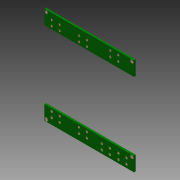
# Autodesk Inventor part: ui_pcb
Saved by Autodesk Inventor 2015 (Build 190159000, 159)
## iProperties
Created: 2014-10-14
Part Number: ui_pcb
Material: Generic
Document SubType Name: Modeling
Designer: Adam
Density: 1 g/cm^3
Appearance: Gold - Metal
Author: Adam
Autodesk Inventor part; units mm, degrees
ref_plane "YZ Plane" through (0, 0, 0) normal (1, 0, 0) x (0, 1, 0)
ref_plane "XZ Plane" through (0, 0, 0) normal (0, 1, 0) x (-1, 0, 0)
ref_plane "Work Plane1" through (0, 0, 0.25) normal (0, 0, 1) x (1, 0, 0)
sketch "Sketch1" plane through (0, 0, 0.25) normal (0, 0, 1) x (1, 0, 0)
  line L0 (4.3349, -0.3556) -> (4.6399, -0.3556) construction
  line L1 (4.6399, -0.3556) -> (4.6399, -1.0668) construction
  line L2 (4.6399, -1.0668) -> (4.3349, -1.0668) construction
  line L3 (4.3349, -1.0668) -> (4.3349, -0.3556) construction
  line L4 (-1.7314, -5.6515) -> (-2.0364, -5.6515) construction
  line L5 (-2.0364, -5.6515) -> (-2.0364, -4.9403) construction
  line L6 (-2.0364, -4.9403) -> (-1.7314, -4.9403) construction
  line L7 (-1.7314, -4.9403) -> (-1.7314, -5.6515) construction
  line L8 (-2.0364, -0.3556) -> (-1.7314, -0.3556) construction
  line L9 (-1.7314, -0.3556) -> (-1.7314, -1.0668) construction
  line L10 (-1.7314, -1.0668) -> (-2.0364, -1.0668) construction
  line L11 (-2.0364, -1.0668) -> (-2.0364, -0.3556) construction
  line L12 (4.3349, -4.9403) -> (4.6399, -4.9403) construction
  line L13 (4.6399, -4.9403) -> (4.6399, -5.6515) construction
  line L14 (4.6399, -5.6515) -> (4.3349, -5.6515) construction
  line L15 (4.3349, -5.6515) -> (4.3349, -4.9403) construction
  line L16 (27.1949, -0.3556) -> (27.4999, -0.3556) construction
  line L17 (27.4999, -0.3556) -> (27.4999, -1.0668) construction
  line L18 (27.4999, -1.0668) -> (27.1949, -1.0668) construction
  line L19 (27.1949, -1.0668) -> (27.1949, -0.3556) construction
  line L20 (21.1286, -5.6515) -> (20.8236, -5.6515) construction
  line L21 (20.8236, -5.6515) -> (20.8236, -4.9403) construction
  line L22 (20.8236, -4.9403) -> (21.1286, -4.9403) construction
  line L23 (21.1286, -4.9403) -> (21.1286, -5.6515) construction
  line L24 (20.8236, -0.3556) -> (21.1286, -0.3556) construction
  line L25 (21.1286, -0.3556) -> (21.1286, -1.0668) construction
  line L26 (21.1286, -1.0668) -> (20.8236, -1.0668) construction
  line L27 (20.8236, -1.0668) -> (20.8236, -0.3556) construction
  line L28 (27.1949, -4.9403) -> (27.4999, -4.9403) construction
  line L29 (27.4999, -4.9403) -> (27.4999, -5.6515) construction
  line L30 (27.4999, -5.6515) -> (27.1949, -5.6515) construction
  line L31 (27.1949, -5.6515) -> (27.1949, -4.9403) construction
  line L32 (46.3349, -2.665) -> (46.6399, -2.665) construction
  line L33 (46.6399, -2.665) -> (46.6399, -3.3762) construction
  line L34 (46.6399, -3.3762) -> (46.3349, -3.3762) construction
  line L35 (46.3349, -3.3762) -> (46.3349, -2.665) construction
  line L36 (40.2686, -7.9609) -> (39.9636, -7.9609) construction
  line L37 (39.9636, -7.9609) -> (39.9636, -7.2497) construction
  line L38 (39.9636, -7.2497) -> (40.2686, -7.2497) construction
  line L39 (40.2686, -7.2497) -> (40.2686, -7.9609) construction
  line L40 (39.9636, -2.665) -> (40.2686, -2.665) construction
  line L41 (40.2686, -2.665) -> (40.2686, -3.3762) construction
  line L42 (40.2686, -3.3762) -> (39.9636, -3.3762) construction
  line L43 (39.9636, -3.3762) -> (39.9636, -2.665) construction
  line L44 (46.3349, -7.2497) -> (46.6399, -7.2497) construction
  line L45 (46.6399, -7.2497) -> (46.6399, -7.9609) construction
  line L46 (46.6399, -7.9609) -> (46.3349, -7.9609) construction
  line L47 (46.3349, -7.9609) -> (46.3349, -7.2497) construction
  line L48 (60.3349, -2.665) -> (60.6399, -2.665) construction
  line L49 (60.6399, -2.665) -> (60.6399, -3.3762) construction
  line L50 (60.6399, -3.3762) -> (60.3349, -3.3762) construction
  line L51 (60.3349, -3.3762) -> (60.3349, -2.665) construction
  line L52 (54.2686, -7.9609) -> (53.9636, -7.9609) construction
  line L53 (53.9636, -7.9609) -> (53.9636, -7.2497) construction
  line L54 (53.9636, -7.2497) -> (54.2686, -7.2497) construction
  line L55 (54.2686, -7.2497) -> (54.2686, -7.9609) construction
  line L56 (53.9636, -2.665) -> (54.2686, -2.665) construction
  line L57 (54.2686, -2.665) -> (54.2686, -3.3762) construction
  line L58 (54.2686, -3.3762) -> (53.9636, -3.3762) construction
  line L59 (53.9636, -3.3762) -> (53.9636, -2.665) construction
  line L60 (60.3349, -7.2497) -> (60.6399, -7.2497) construction
  line L61 (60.6399, -7.2497) -> (60.6399, -7.9609) construction
  line L62 (60.6399, -7.9609) -> (60.3349, -7.9609) construction
  line L63 (60.3349, -7.9609) -> (60.3349, -7.2497) construction
  line L64 (4.3349, 66.082) -> (4.6399, 66.082) construction
  line L65 (4.6399, 66.082) -> (4.6399, 65.3708) construction
  line L66 (4.6399, 65.3708) -> (4.3349, 65.3708) construction
  line L67 (4.3349, 65.3708) -> (4.3349, 66.082) construction
  line L68 (-1.7314, 60.7861) -> (-2.0364, 60.7861) construction
  line L69 (-2.0364, 60.7861) -> (-2.0364, 61.4973) construction
  line L70 (-2.0364, 61.4973) -> (-1.7314, 61.4973) construction
  line L71 (-1.7314, 61.4973) -> (-1.7314, 60.7861) construction
  line L72 (-2.0364, 66.082) -> (-1.7314, 66.082) construction
  line L73 (-1.7314, 66.082) -> (-1.7314, 65.3708) construction
  line L74 (-1.7314, 65.3708) -> (-2.0364, 65.3708) construction
  line L75 (-2.0364, 65.3708) -> (-2.0364, 66.082) construction
  line L76 (4.3349, 61.4973) -> (4.6399, 61.4973) construction
  line L77 (4.6399, 61.4973) -> (4.6399, 60.7861) construction
  line L78 (4.6399, 60.7861) -> (4.3349, 60.7861) construction
  line L79 (4.3349, 60.7861) -> (4.3349, 61.4973) construction
  line L80 (27.1949, 66.082) -> (27.4999, 66.082) construction
  line L81 (27.4999, 66.082) -> (27.4999, 65.3708) construction
  line L82 (27.4999, 65.3708) -> (27.1949, 65.3708) construction
  line L83 (27.1949, 65.3708) -> (27.1949, 66.082) construction
  line L84 (21.1286, 60.7861) -> (20.8236, 60.7861) construction
  line L85 (20.8236, 60.7861) -> (20.8236, 61.4973) construction
  line L86 (20.8236, 61.4973) -> (21.1286, 61.4973) construction
  line L87 (21.1286, 61.4973) -> (21.1286, 60.7861) construction
  line L88 (20.8236, 66.082) -> (21.1286, 66.082) construction
  line L89 (21.1286, 66.082) -> (21.1286, 65.3708) construction
  line L90 (21.1286, 65.3708) -> (20.8236, 65.3708) construction
  line L91 (20.8236, 65.3708) -> (20.8236, 66.082) construction
  line L92 (27.1949, 61.4973) -> (27.4999, 61.4973) construction
  line L93 (27.4999, 61.4973) -> (27.4999, 60.7861) construction
  line L94 (27.4999, 60.7861) -> (27.1949, 60.7861) construction
  line L95 (27.1949, 60.7861) -> (27.1949, 61.4973) construction
  line L96 (47.2686, 63.0955) -> (46.9636, 63.0955) construction
  line L97 (46.9636, 63.0955) -> (46.9636, 63.8067) construction
  line L98 (46.9636, 63.8067) -> (47.2686, 63.8067) construction
  line L99 (47.2686, 63.8067) -> (47.2686, 63.0955) construction
  line L100 (53.3349, 68.3914) -> (53.6399, 68.3914) construction
  line L101 (53.6399, 68.3914) -> (53.6399, 67.6802) construction
  line L102 (53.6399, 67.6802) -> (53.3349, 67.6802) construction
  line L103 (53.3349, 67.6802) -> (53.3349, 68.3914) construction
  line L104 (53.6399, 63.0955) -> (53.3349, 63.0955) construction
  line L105 (53.3349, 63.0955) -> (53.3349, 63.8067) construction
  line L106 (53.3349, 63.8067) -> (53.6399, 63.8067) construction
  line L107 (53.6399, 63.8067) -> (53.6399, 63.0955) construction
  line L108 (47.2686, 67.6802) -> (46.9636, 67.6802) construction
  line L109 (46.9636, 67.6802) -> (46.9636, 68.3914) construction
  line L110 (46.9636, 68.3914) -> (47.2686, 68.3914) construction
  line L111 (47.2686, 68.3914) -> (47.2686, 67.6802) construction
  circle A0 centre (-2.0364, -5.2959) radius 0.5
  circle A1 centre (4.6399, -5.2959) radius 0.5
  circle A2 centre (4.6399, -0.7112) radius 0.5
  circle A3 centre (-2.0364, -0.7112) radius 0.5
  circle A4 centre (20.8236, -0.7112) radius 0.5
  circle A5 centre (20.8236, -5.2959) radius 0.5
  circle A6 centre (27.4999, -5.2959) radius 0.5
  circle A7 centre (27.4999, -0.7112) radius 0.5
  circle A8 centre (39.9636, -3.0206) radius 0.5
  circle A9 centre (39.9636, -7.6053) radius 0.5
  circle A10 centre (46.6399, -3.0206) radius 0.5
  circle A11 centre (46.6399, -7.6053) radius 0.5
  circle A12 centre (53.9636, -3.0206) radius 0.5
  circle A13 centre (53.9636, -7.6053) radius 0.5
  circle A14 centre (60.6399, -3.0206) radius 0.5
  circle A15 centre (60.6399, -7.6053) radius 0.5
  circle A16 centre (-2.0364, 65.7264) radius 0.5
  circle A17 centre (-2.0364, 61.1417) radius 0.5
  circle A18 centre (4.6399, 65.7264) radius 0.5
  circle A19 centre (4.6399, 61.1417) radius 0.5
  circle A20 centre (20.8236, 65.7264) radius 0.5
  circle A21 centre (20.8236, 61.1417) radius 0.5
  circle A22 centre (27.4999, 61.1417) radius 0.5
  circle A23 centre (27.4999, 65.7264) radius 0.5
  circle A24 centre (46.9636, 68.0358) radius 0.5
  circle A25 centre (46.9636, 63.4511) radius 0.5
  circle A26 centre (53.6399, 63.4511) radius 0.5
  circle A27 centre (53.6399, 68.0358) radius 0.5
  line L112 (66.7941, 1.6153) -> (-8.1906, 1.6153)
  line L113 (-8.1906, 1.6153) -> (-8.1906, -10.3847)
  line L114 (-8.1906, -10.3847) -> (66.7941, -10.3847)
  line L115 (66.7941, -10.3847) -> (66.7941, 1.6153)
  line L116 (-8.1906, 58.8153) -> (66.7941, 58.8153)
  line L117 (66.7941, 58.8153) -> (66.7941, 70.8153)
  line L118 (66.7941, 70.8153) -> (-8.1906, 70.8153)
  line L119 (-8.1906, 70.8153) -> (-8.1906, 58.8153)
  line L120 (33.3094, 57.8153) -> (-11.6662, 57.8153) construction
  line L121 (-11.6662, 2.6153) -> (63.2941, 2.6153) construction
  point P0 (0, 0)
  dimension "d1" = 1
  dimension "d4" = 12
  dimension "d5" = 12
  dimension "d10" = 1
  dimension "d11" = 1
  dimension "d12" = 74.9846
  dimension "d13" = 3.4756
  constraints: 240 end point, 58 horizontal, 56 vertical, 28 centre point, 28 midpoint, 27 equal radius, 4 parallel, 2 collinear, 2 perpendicular, 112 other
  measures "d1" diameter of A0
  measures "d4" distance between parallel lines of L112 L114
  measures "d5" distance between parallel lines of L116 L118
  measures "d10" distance between parallel lines of L120 L116
  measures "d11" distance between parallel lines of L121 L112
  measures "d12" distance of L117.end L118.end
  measures "d13" distance from line of L120.end L119
extrude "Extrusion1" add sketch "Sketch1" along normal blind 1.5
sketch "Sketch2" plane through (0, 0, 1.75) normal (0, 0, 1) x (1, 0, 0)
  circle A0 centre (-6.4906, -8.6847) radius 0.75 projected
  circle A1 centre (65.0941, -0.0847) radius 0.75 projected
  circle A2 centre (65.0941, 69.1153) radius 0.75 projected
  circle A3 centre (-6.4906, 69.1153) radius 0.75 projected
  point P0 (0, 0)
extrude "Extrusion2" cut sketch "Sketch2" against normal through all
sketch "Sketch3" plane through (0, 0, 1.75) normal (0, 0, 1) x (1, 0, 0)
  circle A0 centre (65.0941, 69.1153) radius 0.75 projected
  circle A1 centre (-6.4906, 69.1153) radius 0.75 projected
  circle A2 centre (53.6399, 68.0358) radius 0.5 projected
  circle A3 centre (53.6399, 63.4511) radius 0.5 projected
  circle A4 centre (46.9636, 63.4511) radius 0.5 projected
  circle A5 centre (46.9636, 68.0358) radius 0.5 projected
  circle A6 centre (27.4999, 65.7264) radius 0.5 projected
  circle A7 centre (27.4999, 61.1417) radius 0.5 projected
  circle A8 centre (20.8236, 61.1417) radius 0.5 projected
  circle A9 centre (20.8236, 65.7264) radius 0.5 projected
  circle A10 centre (4.6399, 61.1417) radius 0.5 projected
  circle A11 centre (4.6399, 65.7264) radius 0.5 projected
  circle A12 centre (-2.0364, 61.1417) radius 0.5 projected
  circle A13 centre (-2.0364, 65.7264) radius 0.5 projected
  line L0 (-8.1906, 58.8153) -> (66.7941, 58.8153) projected
  line L1 (66.7941, 58.8153) -> (66.7941, 70.8153) projected
  line L2 (66.7941, 70.8153) -> (-8.1906, 70.8153) projected
  line L3 (-8.1906, 70.8153) -> (-8.1906, 58.8153) projected
  circle A14 centre (-6.4906, -8.6847) radius 0.75 projected
  circle A15 centre (65.0941, -0.0847) radius 0.75 projected
  circle A16 centre (60.6399, -7.6053) radius 0.5 projected
  circle A17 centre (60.6399, -3.0206) radius 0.5 projected
  circle A18 centre (53.9636, -7.6053) radius 0.5 projected
  circle A19 centre (53.9636, -3.0206) radius 0.5 projected
  circle A20 centre (46.6399, -7.6053) radius 0.5 projected
  circle A21 centre (46.6399, -3.0206) radius 0.5 projected
  circle A22 centre (39.9636, -7.6053) radius 0.5 projected
  circle A23 centre (39.9636, -3.0206) radius 0.5 projected
  circle A24 centre (27.4999, -0.7112) radius 0.5 projected
  circle A25 centre (27.4999, -5.2959) radius 0.5 projected
  circle A26 centre (20.8236, -5.2959) radius 0.5 projected
  circle A27 centre (20.8236, -0.7112) radius 0.5 projected
  circle A28 centre (-2.0364, -0.7112) radius 0.5 projected
  circle A29 centre (4.6399, -0.7112) radius 0.5 projected
  circle A30 centre (4.6399, -5.2959) radius 0.5 projected
  circle A31 centre (-2.0364, -5.2959) radius 0.5 projected
  line L4 (66.7941, 1.6153) -> (-8.1906, 1.6153) projected
  line L5 (-8.1906, 1.6153) -> (-8.1906, -10.3847) projected
  line L6 (-8.1906, -10.3847) -> (66.7941, -10.3847) projected
  line L7 (66.7941, -10.3847) -> (66.7941, 1.6153) projected
  circle A32 centre (46.9636, 68.0358) radius 1
  circle A33 centre (46.9636, 63.4511) radius 1
  circle A34 centre (53.6399, 63.4511) radius 1
  circle A35 centre (53.6399, 68.0358) radius 1
  circle A36 centre (27.4999, 65.7264) radius 1
  circle A37 centre (27.4999, 61.1417) radius 1
  circle A38 centre (20.8236, 61.1417) radius 1
  circle A39 centre (20.8236, 65.7264) radius 1
  circle A40 centre (4.6399, 65.7264) radius 1
  circle A41 centre (4.6399, 61.1417) radius 1
  circle A42 centre (-2.0364, 61.1417) radius 1
  circle A43 centre (-2.0364, 65.7264) radius 1
  circle A44 centre (60.6399, -3.0206) radius 1
  circle A45 centre (60.6399, -7.6053) radius 1
  circle A46 centre (53.9636, -7.6053) radius 0.5 projected
  circle A47 centre (53.9636, -7.6053) radius 1
  circle A48 centre (53.9636, -3.0206) radius 1
  circle A49 centre (46.6399, -3.0206) radius 0.5 projected
  circle A50 centre (46.6399, -3.0206) radius 1
  circle A51 centre (46.6399, -7.6053) radius 1
  circle A52 centre (39.9636, -7.6053) radius 1
  circle A53 centre (39.9636, -3.0206) radius 1
  circle A54 centre (27.4999, -0.7112) radius 1
  circle A55 centre (27.4999, -5.2959) radius 1
  circle A56 centre (20.8236, -5.2959) radius 1
  circle A57 centre (20.8236, -0.7112) radius 1
  circle A58 centre (4.6399, -0.7112) radius 1
  circle A59 centre (-2.0364, -0.7112) radius 0.5 projected
  circle A60 centre (-2.0364, -0.7112) radius 1
  circle A61 centre (-2.0364, -5.2959) radius 0.5 projected
  circle A62 centre (-2.0364, -5.2959) radius 1
  circle A63 centre (4.6399, -5.2959) radius 1
  circle A64 centre (65.0941, 69.1153) radius 1.5
  circle A65 centre (65.0941, -0.0847) radius 1.5
  circle A66 centre (-6.4906, 69.1153) radius 1.5
  circle A67 centre (-6.4906, -8.6847) radius 1.5
  point P0 (0, 0)
  dimension "d16" = 2
  dimension "d17" = 3
  constraints: 32 centre point, 32 coincident, 30 equal radius
  measures "d16" diameter of A32
  measures "d17" diameter of A66
extrude "Extrusion3" add sketch "Sketch3" along normal blind 0.1 contours A32 | A33 | A34 | A35 | A36 | A37 | A38 | A39 | A40 | A41 | A42 | A43 | A44 | A45 | A47 | A48 | A50 | A51 | A52 | A53 | A54 | A55 | A56 | A57 | A58 | A60 | A62 | A63 | A64 | A65 | A66 | A67
body "Solid1"
